# Autodesk Inventor part: Synchronous Belt
Saved by Autodesk Inventor 2016 (Build 200138000, 138)
## iProperties
Created: 2015-05-16
Part Number: Synchronous Belt
Material: Rubber
Document SubType Name: Modeling
Designer: as
Density: 0.93 g/cm^3
Appearance: Rubber - Black - Version 1.1
Mass: 13.9439 g
Surface Area: 329.855 cm^2
Volume: 14.9934 cm^3
CustomPartVersion: 1
Author: as
Autodesk Inventor part; units mm, degrees
sketch "Sketch Path" plane through (0, 0, 0) normal (0, 0, 1) x (1, 0, 0)
  arc A0 (0, -9.5493) -> (0, 9.5493) centre (0, 0) ccw
  arc A1 (-719.6697, 9.5493) -> (-719.6697, -9.5493) centre (-719.6697, 0) ccw
  line L0 (-719.6697, 9.5493) -> (0, 9.5493)
  line L1 (0, -9.5493) -> (-719.6697, -9.5493)
  constraints: 4 end point, 4 point on circle, 2 centre point
ref_plane "Cross Section Plane" through (0, 9.5493, 0) normal (-1, 0, 0) x (0, 0, 1)
ref_plane "Work Plane2" through (0, 0, 0) normal (-1, 0, 0) x (0, 0, 1)
ref_plane "Work Plane3" through (-719.6697, 0, 0) normal (0.9994, -0.0346, 0) x (0, 0, 1)
sketch "Cross Section" plane through (0, 9.5493, 0) normal (-1, 0, 0) x (0, 0, 1)
  line L0 (-5, 0.5) -> (5, 0.5)
  line L1 (5, 0.5) -> (5, -0.5)
  line L2 (5, -0.5) -> (-5, -0.5)
  line L3 (-5, -0.5) -> (-5, 0.5)
  line L4 (-5, 0) -> (5, 0) construction
  point P0 (0, 0)
  point P1 (0, 0)
  dimension "d0" = 10
  dimension "d4" = 0.5
  dimension "d5" = 0.5
  constraints: 10 end point, 3 midpoint, 2 parallel, 1 coincident, 1 horizontal, 1 perpendicular, 1 other
  measures "d0" distance between parallel lines of L1 L3
  measures "d4" distance between parallel lines of L2 L4
  measures "d5" distance between parallel lines of L4 L0
sweep "Belt" add profiles "Cross Section" path "Sketch Path"
equation "\"d0\" = da_B"
equation "\"d4\" = da_a"
equation "\"d5\" = da_a2"
equation "\"da_B\" = 10"
equation "\"da_pb\" = 5"
equation "\"da_L\" = 1499.33948"
equation "\"da_a\" = 0.5"
equation "\"da_S\" = 2.65"
equation "\"da_Beta\" = 20deg"
equation "\"da_Ht\" = 1.2"
equation "\"da_H\" = 2.2"
equation "\"da_a2\" = 0.5"
body "Solid1"
